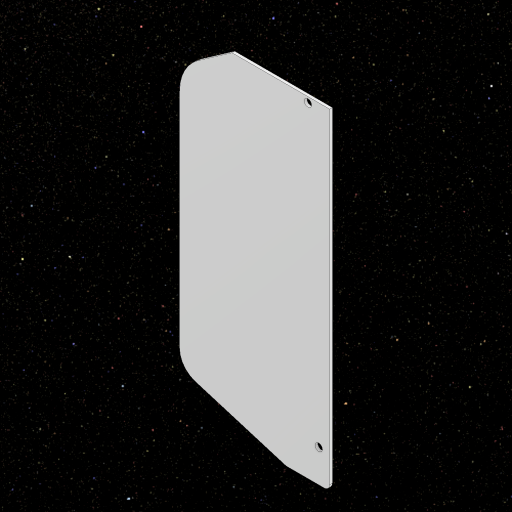
# Autodesk Inventor part: wing
Saved by Autodesk Inventor 2024 (Build 280153000, 153)
## iProperties
Created: 2024-02-14
Part Number: wing
Material: Acetal Resin, White
Document SubType Name: Sheet Metal
Designer: Averey Ku
Density: 1.425 g/cm^3
Sheet Metal Rule: Default
Appearance: Smooth - White
Author: Averey Ku
Autodesk Inventor part; units mm, degrees
ref_plane "YZ Plane" through (0, 0, 0) normal (1, 0, 0) x (0, 1, 0)
ref_plane "XZ Plane" through (0, 0, 0) normal (0, 1, 0) x (-1, 0, 0)
ref_plane "XY Plane" through (0, 0, 0) normal (0, 0, 1) x (1, 0, 0)
sketch "main" plane through (0, 0, 0) normal (0, 0, 1) x (1, 0, 0)
  line L0 (38.5419, -100.052) -> (38.5419, 90.448)
  line L1 (-49.2775, -74.7747) -> (-49.2775, 55.744)
  arc A0 (-49.2775, -74.7747) -> (-40.2846, -86.9216) centre (-36.5775, -74.7747) ccw
  line L2 (13.1419, -103.227) -> (-40.2846, -86.9216)
  circle A1 centre (32.1919, -84.177) radius 2.1844
  line L3 (13.1419, -103.227) -> (35.3669, -103.227)
  arc A2 (35.3669, -103.227) -> (38.5419, -100.052) centre (35.3669, -100.052) ccw
  arc A3 (-38.4463, 76.5505) -> (-49.2775, 55.744) centre (-23.8775, 55.744) ccw
  line L4 (-18.5987, 90.448) -> (-38.4463, 76.5505)
  circle A4 centre (25.8419, 87.273) radius 2.1844
  line L5 (38.5419, 90.448) -> (-18.5987, 90.448)
  point P0 (0.4559, 3.9187)
  point P1 (-49.2775, 68.9664)
  dimension "d3" = 25.4
  dimension "d4" = 12.7
  dimension "d7" = 4.3688
  measures "d3" radius of A3
  measures "d4" radius of A0
  measures "d7" diameter of A4
sketch "Sketch1" plane through (0, 0, 0) normal (0, 0, 1) x (1, 0, 0)
  line L0 (-22.225, -9.525) -> (-22.225, -200.293)
  line L1 (12.7, -200.025) -> (12.7, -9.525)
  line L2 (-75.1194, -174.7477) -> (-75.1194, -44.2289)
  arc A0 (-75.1194, -174.7477) -> (-66.1265, -186.8946) centre (-62.4194, -174.7477) ccw
  line L3 (-12.7, -203.2) -> (-66.1265, -186.8946)
  circle A1 centre (6.35, -184.15) radius 2.1844
  line L4 (-12.7, -203.2) -> (9.525, -203.2)
  arc A2 (9.525, -203.2) -> (12.7, -200.025) centre (9.525, -200.025) ccw
  arc A3 (-64.2882, -23.4225) -> (-75.1194, -44.2289) centre (-49.7194, -44.2289) ccw
  line L5 (-44.4406, -9.525) -> (-64.2882, -23.4225)
  circle A4 centre (0, -12.7) radius 2.1844
  line L6 (12.7, -9.525) -> (-44.4406, -9.525)
  point P0 (0, 0)
  constraints: 2 end point, 1 vertical, 2 other
extrude "Extrusion2" add sketch "Sketch1" along normal blind 1.5875
equation "\"BendRadius\" = Thickness"
equation "\"BendReliefWidth\" = Thickness"
equation "\"BendReliefDepth\" = 0.5 * Thickness"
equation "\"CornerReliefSize\" = 4 * Thickness"
equation "\"MinimumRemnant\" = 2 * Thickness"
equation "\"TransitionRadius\" = BendRadius"
equation "\"JacobiRadiusSize\" = BendRadius"
equation "\"GapSize\" = Thickness"
equation "\"Thickness\" = 3.048"
body "Solid2"
